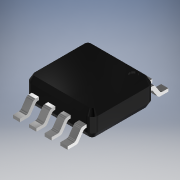
# Autodesk Inventor part: IcNextion
Saved by Autodesk Inventor 2017 SP1 (Build 210196100, 196)
## iProperties
Created: 2016-08-29
Part Number: IcNextion
Material: PBT Plastic
Document SubType Name: Modeling
Designer: jwrjc
Density: 1.31 g/cm^3
Appearance: Smooth - White
Author: jwrjc
Autodesk Inventor part; units mm, degrees
ref_plane "YZ Plane" through (0, 0, 0) normal (1, 0, 0) x (0, 1, 0)
ref_plane "XZ Plane" through (0, 0, 0) normal (0, 1, 0) x (-1, 0, 0)
ref_plane "XY Plane" through (0, 0, 0) normal (0, 0, 1) x (1, 0, 0)
sketch "Sketch1" plane through (0, 0, 0) normal (0, 0, 1) x (1, 0, 0)
  line L0 (-14.0053, 13.8264) -> (-19.3131, 13.8264)
  line L1 (-19.3131, 13.8264) -> (-19.3131, 8.8553)
  line L2 (-19.3131, 8.8553) -> (-14.0053, 8.8553)
  line L3 (-14.0053, 8.8553) -> (-14.0053, 13.8264)
  circle A0 centre (-15.0154, 13.1531) radius 0.2971
  line L4 (-15.0154, 13.8264) -> (-14.441, 13.8264)
  line L5 (-14.441, 13.8264) -> (-14.441, 15.3316)
  line L6 (-14.441, 15.3316) -> (-15.0154, 15.3316)
  line L7 (-15.0154, 15.3316) -> (-15.0154, 13.8264)
  line L8 (-16.2631, 13.8264) -> (-15.7085, 13.8264)
  line L9 (-15.7085, 13.8264) -> (-15.7085, 15.3316)
  line L10 (-15.7085, 15.3316) -> (-16.2631, 15.3316)
  line L11 (-16.2631, 15.3316) -> (-16.2631, 13.8264)
  line L12 (-17.491, 13.8264) -> (-16.9167, 13.8264)
  line L13 (-16.9167, 13.8264) -> (-16.9167, 15.3316)
  line L14 (-16.9167, 15.3316) -> (-17.491, 15.3316)
  line L15 (-17.491, 15.3316) -> (-17.491, 13.8264)
  line L16 (-18.7784, 13.8264) -> (-18.2238, 13.8264)
  line L17 (-18.2238, 13.8264) -> (-18.2238, 15.3316)
  line L18 (-18.2238, 15.3316) -> (-18.7784, 15.3316)
  line L19 (-18.7784, 15.3316) -> (-18.7784, 13.8264)
  line L20 (-14.0053, 11.3409) -> (-19.3131, 11.3409) construction
  line L21 (-14.441, 8.8553) -> (-14.441, 7.3501)
  line L22 (-14.441, 7.3501) -> (-15.0154, 7.3501)
  line L23 (-15.0154, 7.3501) -> (-15.0154, 8.8553)
  line L24 (-15.7085, 8.8553) -> (-15.7085, 7.3501)
  line L25 (-15.7085, 7.3501) -> (-16.2631, 7.3501)
  line L26 (-16.2631, 7.3501) -> (-16.2631, 8.8553)
  line L27 (-16.9167, 8.8553) -> (-16.9167, 7.3501)
  line L28 (-16.9167, 7.3501) -> (-17.491, 7.3501)
  line L29 (-17.491, 7.3501) -> (-17.491, 8.8553)
  line L30 (-18.2238, 8.8553) -> (-18.2238, 7.3501)
  line L31 (-18.2238, 7.3501) -> (-18.7784, 7.3501)
  line L32 (-18.7784, 7.3501) -> (-18.7784, 8.8553)
  line L33 (-14.0053, 8.8553) -> (-19.3131, 8.8553)
  line L34 (-14.441, 8.8553) -> (-14.441, 7.3501)
  line L35 (-14.441, 7.3501) -> (-15.0154, 7.3501)
  line L36 (-15.0154, 7.3501) -> (-15.0154, 8.8553)
  line L37 (-16.2631, 8.8553) -> (-15.7085, 8.8553)
  line L38 (-15.7085, 8.8553) -> (-15.7085, 7.3501)
  line L39 (-15.7085, 7.3501) -> (-16.2631, 7.3501)
  line L40 (-16.2631, 7.3501) -> (-16.2631, 8.8553)
  line L41 (-17.491, 8.8553) -> (-16.9167, 8.8553)
  line L42 (-16.9167, 8.8553) -> (-16.9167, 7.3501)
  line L43 (-16.9167, 7.3501) -> (-17.491, 7.3501)
  line L44 (-17.491, 7.3501) -> (-17.491, 8.8553)
  line L45 (-18.7784, 8.8553) -> (-18.2238, 8.8553)
  line L46 (-18.2238, 8.8553) -> (-18.2238, 7.3501)
  line L47 (-18.2238, 7.3501) -> (-18.7784, 7.3501)
  line L48 (-18.7784, 7.3501) -> (-18.7784, 8.8553)
  line L49 (-14.0053, 8.8553) -> (-19.3131, 8.8553)
  line L50 (-14.441, 8.8553) -> (-14.441, 7.3501)
  line L51 (-14.441, 7.3501) -> (-15.0154, 7.3501)
  line L52 (-15.0154, 7.3501) -> (-15.0154, 8.8553)
  line L53 (-15.0154, 7.3501) -> (-14.441, 7.3501)
  line L54 (-14.441, 7.3501) -> (-14.441, 8.8553)
  line L55 (-14.441, 8.8553) -> (-15.0154, 8.8553)
  line L56 (-15.0154, 8.8553) -> (-15.0154, 7.3501)
  point P0 (0, 0)
  constraints: 114 end point, 18 point on line, 16 symmetric about line, 12 parallel, 6 horizontal, 6 perpendicular, 2 midpoint, 1 centre point
extrude "Extrusion1" add sketch "Sketch1" along normal blind 2 contours L3 L2 L1 L0
extrude "Extrusion2" add sketch "Sketch1" along normal blind 1 separate body contours L0 L7 L6 L5 | L21 L22 L23 L2 | L0 L11 L10 L9 | L24 L25 L26 L2 | L0 L15 L14 L13 | L27 L28 L29 L2 | L0 L19 L18 L17 | L30 L31 L32 L2
fillet "Fillet1" radius 0.5 4 edges at (-19.3131, 13.8264, 1) (-19.3131, 8.8553, 1) (-14.0053, 13.8264, 1) (-14.0053, 8.8553, 1)
chamfer "Chamfer1" distance 0.25 angle 60 9 edges at (-16.6592, 8.8553, 2) (-14.1517, 9.0017, 2) (-14.0053, 11.3409, 2) (-14.1517, 13.68, 2) (-14.7603, 13.8264, 2) (-18.7958, 13.8264, 2) (-19.1667, 13.68, 2) (-19.3131, 11.3409, 2) (-19.1667, 9.0017, 2) measured on face at (-16.1675, 10.2064, 2)
chamfer "Chamfer2" distance 0.25 angle 60 17 edges at (-19.1667, 9.0017, 0) (-16.6592, 8.8553, 0) (-14.1517, 9.0017, 0) (-14.0053, 11.3409, 0) (-14.1517, 13.68, 0) (-14.7603, 13.8264, 0) (-18.7958, 13.8264, 0) (-19.1667, 13.68, 0) (-19.3131, 11.3409, 0) (-15.9858, 8.8553, 0) (-18.5011, 8.8553, 0) (-14.7282, 8.8553, 0) (-17.2039, 8.8553, 0) (-18.5011, 13.8264, 0) (-15.9858, 13.8264, 0) (-17.2039, 13.8264, 0) (-14.7282, 13.8264, 0) measured on face at (-14.6325, 8.8553, 0.3333) measured on face at (-15.8934, 8.8553, 0.3333) measured on face at (-16.0783, 13.8264, 0.3333) measured on face at (-17.1081, 8.8553, 0.3333) measured on face at (-17.2996, 13.8264, 0.3333) measured on face at (-18.4087, 8.8553, 0.3333) measured on face at (-14.8239, 13.8264, 0.3333) measured on face at (-18.5935, 13.8264, 0.3333) measured on face at (-16.1675, 10.2064, 0)
sketch "Sketch2" plane through (-18.7784, 13.8264, 0) normal (-1, 0, 0) x (0, 0, 1)
  line L0 (0, 1.5052) -> (0, 0) projected
  line L1 (0, 1.5052) -> (0.2362, 1.5052)
  line L2 (0, 1.5052) -> (1, 1.5052) projected
  line L3 (0.2362, 0.9081) -> (1, 0.3985)
  line L4 (1, 1.5052) -> (1, 0) projected
  line L5 (1, 0.3985) -> (1, 0)
  line L6 (1, 0) -> (0.7644, 0)
  line L7 (0, 0) -> (1, 0) projected
  line L8 (0.7644, 0.2079) -> (0, 0.7179)
  line L9 (0, 0.7179) -> (0, 1.5052)
  line L10 (0.2362, 1.5052) -> (0.2362, 0.9081)
  line L11 (1, 0.3985) -> (1, 0)
  line L12 (0.7644, 0) -> (0.7644, 0.2079)
  line L13 (1.567, -0.5) -> (1.567, -4.4712) projected
  line L14 (1.567, -2.4856) -> (0.433, -2.4856) construction
  line L15 (0.433, -4.4712) -> (0.433, -0.5) projected
  line L16 (1.567, -2.4856) -> (0.433, -2.4856)
  line L17 (0.2362, 1.5052) -> (1, 1.5052)
  line L18 (0.7644, 0) -> (0, 0)
  line L19 (0, -6.4764) -> (0, -4.9712)
  line L20 (0, -6.4764) -> (1, -6.4764)
  line L21 (0.2362, -5.8793) -> (1, -5.3696)
  line L22 (1, -6.4764) -> (1, -4.9712)
  line L23 (0, -4.9712) -> (1, -4.9712)
  line L24 (0.7644, -5.179) -> (0, -5.6891)
  line L25 (0.2362, -6.4764) -> (0.2362, -5.8793)
  line L26 (0.7644, -4.9712) -> (0.7644, -5.179)
  line L27 (0.7644, -4.9712) -> (0.7644, -5.179)
  line L28 (0, -5.6891) -> (0, -4.9712)
  line L29 (1, -5.3696) -> (1, -6.4764)
  line L30 (0.2362, -6.4764) -> (0.2362, -5.8793)
  point P0 (0, -13.8264)
  constraints: 50 end point, 10 symmetric about line, 6 collinear, 4 parallel, 4 point on line, 2 midpoint, 1 horizontal, 1 perpendicular, 1 vertical
extrude "Extrusion3" cut sketch "Sketch2" against normal blind 4.5 contours L8 L12 L7 L0 | L2 L4 L3 L10 | L19 L23 L26 L24 | L25 L21 L22 L20 bodies 2
fillet "Fillet2" radius 0.25 32 edges at (-14.7282, 14.2249, 1) (-15.9858, 14.2249, 1) (-17.2039, 14.2249, 1) (-18.5011, 14.2249, 1) (-18.5011, 8.4568, 1) (-17.2039, 8.4568, 1) (-15.9858, 8.4568, 1) (-14.7282, 8.4568, 1) (-14.7282, 7.9472, 0.2362) (-15.9858, 7.9472, 0.2362) (-17.2039, 7.9472, 0.2362) (-18.5011, 7.9472, 0.2362) (-18.5011, 14.7346, 0.2362) (-17.2039, 14.7346, 0.2362) (-15.9858, 14.7346, 0.2362) (-14.7282, 14.7346, 0.2362) (-18.5011, 14.0343, 0.7644) (-17.2039, 14.0343, 0.7644) (-15.9858, 14.0343, 0.7644) (-14.7282, 14.0343, 0.7644) (-14.7282, 14.5443, 0) (-15.9858, 14.5443, 0) (-17.2039, 14.5443, 0) (-18.5011, 14.5443, 0) (-18.5011, 8.6474, 0.7644) (-18.5011, 8.1374, 0) (-17.2039, 8.1374, 0) (-17.2039, 8.6474, 0.7644) (-15.9858, 8.6474, 0.7644) (-15.9858, 8.1374, 0) (-14.7282, 8.1374, 0) (-14.7282, 8.6474, 0.7644)
extrude "Extrusion4" add sketch "Sketch1" along normal blind 1.85 separate body contours A0
body "Solid1"
body "Solid2"
body "Solid3"
